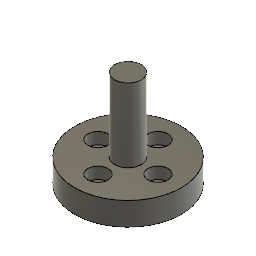
Spinner (Autodesk Fusion 360 design; units mm, degrees)
Autodesk Fusion 360 part; units mm, degrees
note: some values were not read from the file. Set by a fixed rule: which sketch regions a step uses.
sketch "Sketch1" plane through (0, 0, 0) normal (0, 0, 1) x (1, 0, 0)
  line L0 (0, 0) -> (8, 0)
  line L1 (8, 0) -> (8, 3.5)
  line L2 (8, 3.5) -> (2, 3.5)
  line L3 (2, 3.5) -> (2, 14.5)
  line L4 (2, 14.5) -> (0, 14.5)
  line L5 (0, 14.5) -> (0, 0)
  constraint coincident L0.start L5.end
  constraint horizontal L0
  constraint perpendicular L0 L1
  constraint perpendicular L1 L2
  constraint perpendicular L2 L3
  constraint perpendicular L3 L4
  constraint perpendicular L0 L5
revolve "Revolve1" add sketch "Sketch1" angle 360 about axis through (0, 14.5, 0) along (0, -1, 0)
sketch "Sketch2" plane through (0, 3.5, 0) normal (0, 1, 0) x (-1, 0, 0)
  circle A0 centre (0, 0) radius 2
  circle A1 centre (0, 0) radius 8
  circle A2 centre (0, 0) radius 4.5
  line L0 (0, 0) -> (1, 0) construction
  line L1 (1, 0) -> (8, 0) construction
  line L2 (0, 0) -> (0, -0.385) construction
  line L3 (0, -0.385) -> (0, -8) construction
  line L4 (0, 0) -> (-8, 0) construction
  line L5 (0, 0) -> (0, 8) construction
  circle A3 centre (4.5, 0) radius 1.5
  constraint coincident A0.centre A1.centre
  constraint horizontal L0
  constraint coincident A1 L1.end
  constraint parallel L0 L1
  constraint perpendicular L0 L2
  constraint coincident A1 L3.end
  constraint perpendicular L0 L3
  constraint coincident A1 L4.end
  constraint perpendicular L2 L4
  constraint coincident A1 L5.end
  constraint parallel L2 L5
  constraint midpoint L1 A3.centre
extrude "Extrude1" cut sketch "Sketch2" against normal blind 1.75 contours A2 A3 | A2 A3 picked at (4.0029, -0.277) picked at (4.9442, -0.3776)
sketch "Sketch3" plane through (0, 1.75, 0) normal (0, 1, 0) x (-1, 0, 0)
  circle A0 centre (4.5, 0) radius 1.5
  circle A1 centre (4.5, 0) radius 0.75
  dimension "d10" = 1.5
  constraint concentric A0 A1
  measures "d10" diameter of A1
extrude "Extrude2" cut sketch "Sketch3" against normal blind 5 contours A1
pattern_circular "C-Pattern1" count 4 over 360 about axis through (0, 1.75, 0) along (0, 1, 0) of "Extrude1"
pattern_circular "C-Pattern2" count 4 over 360 about axis through (0, 1.75, 0) along (0, 1, 0) of "Extrude2"
